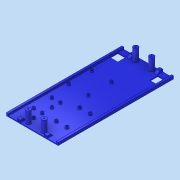
# Autodesk Inventor part: raspi_board_tray
Saved by Autodesk Inventor 2022 (Build 260153000, 153)
## iProperties
Created: 2020-11-04
Part Number: raspi_board_tray
Material: Generic
Document SubType Name: Modeling
Designer: nnico
Density: 1 g/cm^3
Appearance: Blue - Wall Paint - Glossy
Author: nnico
Autodesk Inventor part; units mm, degrees
ref_plane "YZ Plane" through (0, 0, 0) normal (1, 0, 0) x (0, 1, 0)
ref_plane "XZ Plane" through (0, 0, 0) normal (0, 1, 0) x (-1, 0, 0)
ref_plane "XY Plane" through (0, 0, 0) normal (0, 0, 1) x (1, 0, 0)
sketch "Sketch1" plane through (0, 0, 0) normal (0, 1, 0) x (-1, 0, 0)
  line L0 (65, -145) -> (-65, -145)
  line L1 (-65, -145) -> (-65, 145)
  line L2 (-65, 145) -> (65, 145)
  line L3 (65, 145) -> (65, -145)
  line L4 (65, 0) -> (-65, 0) construction
  line L5 (0, -145) -> (0, 145) construction
  point P0 (0, 0)
  point P1 (0, 0)
  dimension "d0" = 130
  dimension "d1" = 290
  constraints: 12 end point, 5 midpoint, 2 parallel, 1 coincident, 1 horizontal, 1 perpendicular
  measures "d0" distance of L1.end L2.end
  measures "d1" distance of L0.end L1.end
extrude "Extrusion1" add sketch "Sketch1" along normal blind 2
sketch "Sketch2" plane through (0, 0, 0) normal (0, -1, 0) x (1, 0, 0)
  line L0 (65, -145) -> (-65, -145) construction
  line L1 (0, -145) -> (0, 145) construction
  line L2 (-65, 145) -> (65, 145) construction
  line L3 (65, 145) -> (65, -145) construction
  line L4 (65, 0) -> (-65, 0) construction
  line L5 (-65, -145) -> (-65, 145) construction
  line L6 (-38, -145) -> (-30, -145)
  line L7 (-30, -145) -> (-30, -131)
  line L8 (-30, -131) -> (-38, -131)
  line L9 (-38, -131) -> (-38, -145)
  line L10 (38, -145) -> (30, -145)
  line L11 (30, -145) -> (30, -131)
  line L12 (30, -131) -> (38, -131)
  line L13 (38, -131) -> (38, -145)
  line L14 (-38, 145) -> (-30, 145)
  line L15 (-30, 145) -> (-30, 131)
  line L16 (-30, 131) -> (-38, 131)
  line L17 (-38, 131) -> (-38, 145)
  line L18 (30, 145) -> (30, 131)
  line L19 (38, 131) -> (38, 145)
  line L20 (30, 131) -> (38, 131)
  line L21 (38, 145) -> (30, 145)
  point P0 (0, 0)
  dimension "d4" = 8
  dimension "d5" = 14
  dimension "d6" = 30
  constraints: 36 end point, 12 symmetric about line, 4 midpoint, 2 parallel, 1 horizontal, 1 perpendicular, 1 point on line
  measures "d4" distance of L8.end L7.end
  measures "d5" distance of L7.end L6.end
  measures "d6" distance of L6.end L1.start
extrude "Extrusion2" add sketch "Sketch2" against normal blind 8
chamfer "Chamfer1" distance 6 angle 45 4 edges at (-34, 8, 131) (34, 8, 131) (-34, 8, -131) (34, 8, -131)
sketch "Sketch3" plane through (65, 0, -145) normal (0, 0, -1) x (-1, 0, 0)
  line L0 (65, 0) -> (65, 2) construction
  line L1 (35, 2) -> (95, 2) construction
  circle A0 centre (31, 4) radius 1.75
  line L2 (27, 8) -> (35, 8) projected
  line L3 (35, 2) -> (35, 8) projected
  circle A1 centre (99, 4) radius 1.75
  dimension "d12" = 3.5
  dimension "d13" = 4
  dimension "d14" = 4
  constraints: 2 centre point, 2 end point, 1 midpoint, 1 symmetric about line, 1 other
  measures "d12" diameter of A0
  measures "d13" distance from line of L2 A0.centre
  measures "d14" distance from line of L3 A0.centre
extrude "Extrusion3" cut sketch "Sketch3" against normal blind 6
sketch "Sketch4" plane through (-65, 0, 145) normal (0, 0, 1) x (1, 0, 0)
  circle A0 centre (99, 4) radius 1.75 projected
  circle A1 centre (31, 4) radius 1.75 projected
  point P0 (65, 0)
extrude "Extrusion4" cut sketch "Sketch4" against normal blind 6
sketch "Sketch5" plane through (0, 2, 0) normal (0, 1, 0) x (1, 0, 0)
  line L0 (-60, 130) -> (-40, 130)
  line L1 (-40, 130) -> (-40, 110)
  line L2 (-40, 110) -> (-60, 110)
  line L3 (-60, 110) -> (-60, 130)
  line L4 (-38, 145) -> (-65, 145) projected
  line L5 (-65, 145) -> (-65, -145) projected
  line L6 (-65, 145) -> (65, 145) construction
  line L7 (0, 145) -> (0, -145) construction
  line L8 (-30, -145) -> (30, -145) construction
  line L9 (60, 130) -> (40, 130)
  line L10 (40, 130) -> (40, 110)
  line L11 (40, 110) -> (60, 110)
  line L12 (60, 110) -> (60, 130)
  point P0 (0, 0)
  dimension "d19" = 20
  dimension "d20" = 20
  dimension "d21" = 15
  dimension "d22" = 5
  constraints: 18 end point, 4 symmetric about line, 2 midpoint, 2 parallel, 1 horizontal, 1 perpendicular
  measures "d19" distance of L1.end L2.end
  measures "d20" distance of L0.end L1.end
  measures "d21" distance from line of L4 L0.start
  measures "d22" distance between parallel lines of L5 L3
extrude "Extrusion5" cut sketch "Sketch5" against normal up to next
sketch "Sketch6" plane through (0, 2, 0) normal (0, 1, 0) x (1, 0, 0)
  line L0 (-51.5, -1.5) -> (-2.5, -1.5) construction
  line L1 (-2.5, -1.5) -> (-2.5, 56.5) construction
  line L2 (-2.5, 56.5) -> (-51.5, 56.5) construction
  line L3 (-51.5, 56.5) -> (-51.5, -1.5) construction
  line L4 (65, -145) -> (-65, -145) construction
  line L5 (-65, 145) -> (65, 145) construction
  line L6 (-27, -1.5) -> (-27, 56.5) construction
  line L7 (-40, 110) -> (-60, 110) construction
  line L8 (-55, -5) -> (1, -5) construction
  line L9 (1, -5) -> (1, 80) construction
  line L10 (1, 80) -> (-55, 80) construction
  line L11 (-55, 80) -> (-55, -5) construction
  circle A0 centre (-2.5, -1.5) radius 1.75
  circle A1 centre (-51.5, -1.5) radius 1.75
  circle A2 centre (-51.5, 56.5) radius 1.75
  circle A3 centre (-2.5, 56.5) radius 1.75
  circle A4 centre (-2.5, -1.5) radius 3.5
  circle A5 centre (-2.5, 56.5) radius 3.5
  circle A6 centre (-51.5, -1.5) radius 3.5
  circle A7 centre (-51.5, 56.5) radius 3.5
  line L12 (-65, 145) -> (-65, -145) projected
  point P0 (0, 0)
  dimension "d25" = 49
  dimension "d26" = 58
  dimension "d28" = 56
  dimension "d29" = 85
  dimension "d30" = 3.5
  dimension "d31" = 3.5
  dimension "d32" = 30
  dimension "d33" = 3.5
  dimension "d34" = 3.5
  dimension "d35" = 3.5
  dimension "d36" = 3.5
  dimension "d79" = 10
  constraints: 18 end point, 8 centre point, 8 coincident, 4 parallel, 3 tangent, 2 horizontal, 2 midpoint, 2 perpendicular
  measures "d25" distance of L2.end L1.end
  measures "d26" distance of L1.end L0.end
  measures "d28" distance of L10.end L9.end
  measures "d29" distance of L9.end L8.end
  measures "d30" horizontal distance of L8.end L0.end
  measures "d31" horizontal distance of L0.end L8.end
  measures "d32" vertical distance of L7.start L10.end
  measures "d33" diameter of A0
  measures "d34" diameter of A1
  measures "d35" diameter of A2
  measures "d36" diameter of A3
  measures "d79" distance from line of L12 L10.end
extrude "Extrusion6" add sketch "Sketch6" along normal blind 4
sketch "Sketch7" plane through (0, 2, 0) normal (0, 1, 0) x (1, 0, 0)
  line L0 (-45.4, -121) -> (-20, -121) construction
  line L1 (-20, -121) -> (-20, -50.2) construction
  line L2 (-20, -50.2) -> (-45.4, -50.2) construction
  line L3 (-45.4, -50.2) -> (-45.4, -121) construction
  line L4 (-30, -145) -> (30, -145) construction
  line L5 (30, 145) -> (-30, 145) construction
  line L6 (-38, -131) -> (-30, -131) construction
  line L7 (-20, -121) -> (-45.4, -121) construction
  line L8 (-45.4, -121) -> (-45.4, -95.6) construction
  line L9 (-45.4, -95.6) -> (-20, -95.6) construction
  line L10 (-20, -95.6) -> (-20, -121) construction
  line L11 (-45.4, -75.6) -> (-20, -75.6) construction
  line L12 (-20, -75.6) -> (-20, -50.2) construction
  line L13 (-20, -50.2) -> (-45.4, -50.2) construction
  line L14 (-45.4, -50.2) -> (-45.4, -75.6) construction
  line L15 (-20, -108.3) -> (-45.4, -108.3) construction
  line L16 (-43.241, -118.841) -> (-22.159, -118.841) construction
  line L17 (-22.159, -118.841) -> (-22.159, -97.759) construction
  line L18 (-22.159, -97.759) -> (-43.241, -97.759) construction
  line L19 (-43.241, -97.759) -> (-43.241, -118.841) construction
  line L20 (-43.241, -108.3) -> (-22.159, -108.3) construction
  line L21 (-32.7, -118.841) -> (-32.7, -97.759) construction
  circle A0 centre (-43.241, -97.759) radius 1.75
  circle A1 centre (-43.241, -97.759) radius 3.5
  circle A2 centre (-22.159, -97.759) radius 1.75
  circle A3 centre (-22.159, -97.759) radius 3.5
  circle A4 centre (-22.159, -118.841) radius 1.75
  circle A5 centre (-22.159, -118.841) radius 3.5
  line L22 (-43.241, -73.441) -> (-22.159, -73.441) construction
  line L23 (-22.159, -73.441) -> (-22.159, -52.359) construction
  line L24 (-22.159, -52.359) -> (-43.241, -52.359) construction
  line L25 (-43.241, -52.359) -> (-43.241, -73.441) construction
  line L26 (-43.241, -62.9) -> (-22.159, -62.9) construction
  line L27 (-32.7, -73.441) -> (-32.7, -52.359) construction
  circle A6 centre (-43.241, -52.359) radius 3.5
  circle A7 centre (-43.241, -52.359) radius 1.75
  circle A8 centre (-22.159, -52.359) radius 3.5
  circle A9 centre (-22.159, -52.359) radius 1.75
  circle A10 centre (-22.159, -73.441) radius 3.5
  circle A11 centre (-22.159, -73.441) radius 1.75
  line L28 (-45.4, -62.9) -> (-20, -62.9) construction
  line L29 (65, -145) -> (-65, -145) construction
  line L30 (0, -145) -> (0, 145) construction
  point P0 (0, 0)
  point P1 (-32.7, -108.3)
  point P2 (-32.7, -62.9)
  dimension "d39" = 25.4
  dimension "d40" = 10
  dimension "d41" = 25.4
  dimension "d42" = 25.4
  dimension "d57" = 21.082
  dimension "d58" = 21.082
  dimension "d61" = 3.5
  dimension "d62" = 7
  dimension "d63" = 3.5
  dimension "d64" = 7
  dimension "d65" = 3.5
  dimension "d66" = 7
  dimension "d67" = 21.082
  dimension "d68" = 21.082
  dimension "d71" = 3.5
  dimension "d72" = 7
  dimension "d73" = 3.5
  dimension "d74" = 7
  dimension "d76" = 7
  dimension "d91" = 20
  dimension "d92" = 20
  constraints: 54 end point, 18 midpoint, 12 centre point, 12 coincident, 10 parallel, 5 horizontal, 5 perpendicular, 3 point on line, 1 collinear
  measures "d39" distance of L2.end L1.end
  measures "d40" distance from line of L0.start L6
  measures "d41" distance of L7.end L8.end
  measures "d42" distance of L12.end L11.end
  measures "d57" distance of L18.end L17.end
  measures "d58" distance of L17.end L16.end
  measures "d61" diameter of A0
  measures "d62" diameter of A1
  measures "d63" diameter of A2
  measures "d64" diameter of A3
  measures "d65" diameter of A4
  measures "d66" diameter of A5
  measures "d67" distance of L25.start L23.end
  measures "d68" distance of L23.end L22.end
  measures "d71" diameter of A7
  measures "d72" diameter of A6
  measures "d73" diameter of A9
  measures "d74" diameter of A8
  measures "d76" diameter of A10
  measures "d91" distance between parallel lines of L30 L1
  measures "d92" distance between parallel lines of L11 L9
extrude "Extrusion7" add sketch "Sketch7" along normal blind 4
sketch "Sketch8" plane through (0, 2, 0) normal (0, 1, 0) x (1, 0, 0)
  line L0 (-65, 145) -> (65, 145) construction
  line L1 (0, 145) -> (0, -145) construction
  line L2 (-30, -145) -> (30, -145) construction
  line L3 (-65, -145) -> (-65, 145) construction
  line L4 (-65, 0) -> (65, 0) construction
  line L5 (65, 145) -> (65, -145) construction
  circle A0 centre (-20, 135) radius 6
  circle A1 centre (20, 135) radius 6
  circle A2 centre (-20, -135) radius 6
  circle A3 centre (20, -135) radius 6
  point P0 (0, 0)
  dimension "d80" = 12
  dimension "d81" = 10
  dimension "d82" = 40
  constraints: 4 centre point, 4 end point, 4 midpoint, 3 symmetric about line, 3 other
  measures "d80" diameter of A0
  measures "d81" distance from line of L0 A0.centre
  measures "d82" diameter of A0.centre L1
extrude "Extrusion8" add sketch "Sketch8" along normal blind 30
sketch "Sketch9" plane through (-20, 32, 135) normal (0, 1, 0) x (1, 0, 0)
  circle A0 centre (0, 0) radius 6 projected
  circle A1 centre (40, 0) radius 6 projected
  circle A2 centre (0, 270) radius 6 projected
  circle A3 centre (40, 270) radius 6 projected
  line L0 (-45, 280) -> (-45, -10) construction
  line L1 (-45, 135) -> (85, 135) construction
  line L2 (85, -10) -> (85, 280) construction
  line L3 (-45, 280) -> (85, 280) construction
  line L4 (20, 280) -> (20, -10) construction
  line L5 (-10, -10) -> (50, -10) construction
  circle A4 centre (0, 270) radius 1.625
  circle A5 centre (40, 270) radius 1.625
  circle A6 centre (0, 0) radius 1.625
  circle A7 centre (40, 0) radius 1.625
  point P0 (20, 135)
  dimension "d85" = 3.25
  constraints: 4 centre point, 4 end point, 4 midpoint, 3 symmetric about line, 1 coincident, 3 other
  measures "d85" diameter of A4
extrude "Extrusion9" cut sketch "Sketch9" against normal blind 10 contours A4 | A5 | A6 | A7
sketch "Sketch10" plane through (0, 2, 0) normal (0, 1, 0) x (1, 0, 0)
  line L0 (65, -145) -> (-65, -145) construction
  line L1 (0, -145) -> (0, 145) construction
  line L2 (-65, 145) -> (65, 145) construction
  line L3 (65, -145) -> (60, -145)
  line L4 (60, -145) -> (60, 145)
  line L5 (60, 145) -> (65, 145)
  line L6 (65, 145) -> (65, -145)
  line L7 (-65, -145) -> (-60, -145)
  line L8 (-60, -145) -> (-60, 145)
  line L9 (-60, 145) -> (-65, 145)
  line L10 (-65, 145) -> (-65, -145)
  point P0 (0, 0)
  point P1 (-65, 145)
  constraints: 18 end point, 4 symmetric about line, 2 midpoint, 2 parallel, 1 horizontal, 1 perpendicular, 1 point on line
extrude "Extrusion10" add sketch "Sketch10" along normal blind 5
sketch "Sketch11" plane through (0, 2, 0) normal (0, 1, 0) x (1, 0, 0)
  line L0 (13.5, -97.75) -> (40, -97.75) construction
  line L1 (40, -97.75) -> (40, -39.25) construction
  line L2 (40, -39.25) -> (13.5, -39.25) construction
  line L3 (13.5, -39.25) -> (13.5, -97.75) construction
  line L4 (60, 145) -> (60, -145) construction
  line L5 (3.75, -101) -> (49.75, -101) construction
  line L6 (49.75, -101) -> (49.75, -36) construction
  line L7 (49.75, -36) -> (3.75, -36) construction
  line L8 (3.75, -36) -> (3.75, -101) construction
  line L9 (26.75, -97.75) -> (26.75, -39.25) construction
  line L10 (13.5, -68.5) -> (40, -68.5) construction
  line L11 (30, -131) -> (38, -131) construction
  circle A0 centre (13.5, -97.75) radius 2.25
  circle A1 centre (13.5, -97.75) radius 4
  circle A2 centre (13.5, -39.25) radius 2.25
  circle A3 centre (13.5, -39.25) radius 4
  circle A4 centre (40, -39.25) radius 2.25
  circle A5 centre (40, -39.25) radius 4
  circle A6 centre (40, -97.75) radius 2.25
  circle A7 centre (40, -97.75) radius 4
  point P0 (0, 0)
  dimension "d93" = 26.5
  dimension "d94" = 58.5
  dimension "d95" = 20
  dimension "d96" = 46
  dimension "d97" = 65
  dimension "d98" = 30
  dimension "d99" = 4.5
  dimension "d100" = 8
  dimension "d101" = 4.5
  dimension "d102" = 8
  dimension "d103" = 4.5
  dimension "d104" = 8
  dimension "d105" = 4.5
  dimension "d106" = 8
  constraints: 20 end point, 8 centre point, 5 coincident, 4 midpoint, 4 parallel, 2 horizontal, 2 perpendicular, 2 other
  measures "d93" distance of L0.start L0.end
  measures "d94" distance of L2.end L0.start
  measures "d95" distance from line of L4 L0.end
  measures "d96" distance of L5.start L5.end
  measures "d97" distance of L7.end L5.start
  measures "d98" distance between parallel lines of L5 L11
  measures "d99" diameter of A0
  measures "d100" diameter of A1
  measures "d101" diameter of A2
  measures "d102" diameter of A3
  measures "d103" diameter of A4
  measures "d104" diameter of A5
  measures "d105" diameter of A6
  measures "d106" diameter of A7
extrude "Extrusion11" add sketch "Sketch11" along normal blind 4
body "Solid1"
